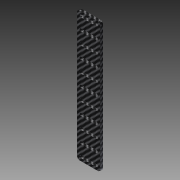
# Autodesk Inventor part: Kicker Plate
Saved by Autodesk Inventor 2015 (Build 190159000, 159)
## iProperties
Created: 2016-09-23
Part Number: Kicker Plate
Material: Generic
Document SubType Name: Modeling
Designer: James Yelland
Density: 1 g/cm^3
Appearance: Default
Author: James Yelland
Autodesk Inventor part; units mm, degrees
ref_plane "YZ Plane" through (0, 0, 0) normal (1, 0, 0) x (0, 1, 0)
ref_plane "XZ Plane" through (0, 0, 0) normal (0, 1, 0) x (-1, 0, 0)
ref_plane "XY Plane" through (0, 0, 0) normal (0, 0, 1) x (1, 0, 0)
sketch "Sketch1" plane through (0, 0, 0) normal (0, 1, 0) x (-1, 0, 0)
  line L0 (-9, 48) -> (-9, -48)
  line L1 (-7, -50) -> (7, -50)
  line L2 (9, -48) -> (9, 48)
  line L3 (7, 50) -> (-7, 50)
  line L4 (-9, 50) -> (9, -50) construction
  line L5 (-9, -50) -> (9, 50) construction
  arc A0 (9, 48) -> (7, 50) centre (7, 48) ccw
  arc A1 (-7, 50) -> (-9, 48) centre (-7, 48) ccw
  arc A2 (-9, -48) -> (-7, -50) centre (-7, -48) ccw
  arc A3 (7, -50) -> (9, -48) centre (7, -48) ccw
  line L6 (-7, 47) -> (-7, 47)
  line L7 (-6, 46) -> (6, 46)
  line L8 (7, 47) -> (7, 47)
  line L9 (6, 48) -> (-6, 48)
  arc A4 (7, 47) -> (6, 48) centre (6, 47) ccw
  arc A5 (6, 46) -> (7, 47) centre (6, 47) ccw
  arc A6 (-6, 48) -> (-7, 47) centre (-6, 47) ccw
  arc A7 (-7, 47) -> (-6, 46) centre (-6, 47) ccw
  line L10 (-7, 37.6) -> (-7, 37.6)
  line L11 (-6, 36.6) -> (6, 36.6)
  line L12 (7, 37.6) -> (7, 37.6)
  line L13 (6, 38.6) -> (-6, 38.6)
  arc A8 (7, 37.6) -> (6, 38.6) centre (6, 37.6) ccw
  arc A9 (6, 36.6) -> (7, 37.6) centre (6, 37.6) ccw
  arc A10 (-6, 38.6) -> (-7, 37.6) centre (-6, 37.6) ccw
  arc A11 (-7, 37.6) -> (-6, 36.6) centre (-6, 37.6) ccw
  line L14 (-7, 28.2) -> (-7, 28.2)
  line L15 (-6, 27.2) -> (6, 27.2)
  line L16 (7, 28.2) -> (7, 28.2)
  line L17 (6, 29.2) -> (-6, 29.2)
  arc A12 (7, 28.2) -> (6, 29.2) centre (6, 28.2) ccw
  arc A13 (6, 27.2) -> (7, 28.2) centre (6, 28.2) ccw
  arc A14 (-6, 29.2) -> (-7, 28.2) centre (-6, 28.2) ccw
  arc A15 (-7, 28.2) -> (-6, 27.2) centre (-6, 28.2) ccw
  line L18 (-7, 18.8) -> (-7, 18.8)
  line L19 (-6, 17.8) -> (6, 17.8)
  line L20 (7, 18.8) -> (7, 18.8)
  line L21 (6, 19.8) -> (-6, 19.8)
  arc A16 (7, 18.8) -> (6, 19.8) centre (6, 18.8) ccw
  arc A17 (6, 17.8) -> (7, 18.8) centre (6, 18.8) ccw
  arc A18 (-6, 19.8) -> (-7, 18.8) centre (-6, 18.8) ccw
  arc A19 (-7, 18.8) -> (-6, 17.8) centre (-6, 18.8) ccw
  line L22 (-7, 9.4) -> (-7, 9.4)
  line L23 (-6, 8.4) -> (6, 8.4)
  line L24 (7, 9.4) -> (7, 9.4)
  line L25 (6, 10.4) -> (-6, 10.4)
  arc A20 (7, 9.4) -> (6, 10.4) centre (6, 9.4) ccw
  arc A21 (6, 8.4) -> (7, 9.4) centre (6, 9.4) ccw
  arc A22 (-6, 10.4) -> (-7, 9.4) centre (-6, 9.4) ccw
  arc A23 (-7, 9.4) -> (-6, 8.4) centre (-6, 9.4) ccw
  line L26 (-7, 0) -> (-7, 0)
  line L27 (-6, -1) -> (6, -1)
  line L28 (7, 0) -> (7, 0)
  line L29 (6, 1) -> (-6, 1)
  arc A24 (7, 0) -> (6, 1) centre (6, 0) ccw
  arc A25 (6, -1) -> (7, 0) centre (6, 0) ccw
  arc A26 (-6, 1) -> (-7, 0) centre (-6, 0) ccw
  arc A27 (-7, 0) -> (-6, -1) centre (-6, 0) ccw
  line L30 (-7, -9.4) -> (-7, -9.4)
  line L31 (-6, -10.4) -> (6, -10.4)
  line L32 (7, -9.4) -> (7, -9.4)
  line L33 (6, -8.4) -> (-6, -8.4)
  arc A28 (7, -9.4) -> (6, -8.4) centre (6, -9.4) ccw
  arc A29 (6, -10.4) -> (7, -9.4) centre (6, -9.4) ccw
  arc A30 (-6, -8.4) -> (-7, -9.4) centre (-6, -9.4) ccw
  arc A31 (-7, -9.4) -> (-6, -10.4) centre (-6, -9.4) ccw
  line L34 (-7, -18.8) -> (-7, -18.8)
  line L35 (-6, -19.8) -> (6, -19.8)
  line L36 (7, -18.8) -> (7, -18.8)
  line L37 (6, -17.8) -> (-6, -17.8)
  arc A32 (7, -18.8) -> (6, -17.8) centre (6, -18.8) ccw
  arc A33 (6, -19.8) -> (7, -18.8) centre (6, -18.8) ccw
  arc A34 (-6, -17.8) -> (-7, -18.8) centre (-6, -18.8) ccw
  arc A35 (-7, -18.8) -> (-6, -19.8) centre (-6, -18.8) ccw
  line L38 (-7, -28.2) -> (-7, -28.2)
  line L39 (-6, -29.2) -> (6, -29.2)
  line L40 (7, -28.2) -> (7, -28.2)
  line L41 (6, -27.2) -> (-6, -27.2)
  arc A36 (7, -28.2) -> (6, -27.2) centre (6, -28.2) ccw
  arc A37 (6, -29.2) -> (7, -28.2) centre (6, -28.2) ccw
  arc A38 (-6, -27.2) -> (-7, -28.2) centre (-6, -28.2) ccw
  arc A39 (-7, -28.2) -> (-6, -29.2) centre (-6, -28.2) ccw
  line L42 (-7, -37.6) -> (-7, -37.6)
  line L43 (-6, -38.6) -> (6, -38.6)
  line L44 (7, -37.6) -> (7, -37.6)
  line L45 (6, -36.6) -> (-6, -36.6)
  arc A40 (7, -37.6) -> (6, -36.6) centre (6, -37.6) ccw
  arc A41 (6, -38.6) -> (7, -37.6) centre (6, -37.6) ccw
  arc A42 (-6, -36.6) -> (-7, -37.6) centre (-6, -37.6) ccw
  arc A43 (-7, -37.6) -> (-6, -38.6) centre (-6, -37.6) ccw
  line L46 (-7, -47) -> (-7, -47)
  line L47 (-6, -48) -> (6, -48)
  line L48 (7, -47) -> (7, -47)
  line L49 (6, -46) -> (-6, -46)
  arc A44 (7, -47) -> (6, -46) centre (6, -47) ccw
  arc A45 (6, -48) -> (7, -47) centre (6, -47) ccw
  arc A46 (-6, -46) -> (-7, -47) centre (-6, -47) ccw
  arc A47 (-7, -47) -> (-6, -48) centre (-6, -47) ccw
  point P0 (0, 0)
  point P1 (-7, 46)
  point P2 (7, 38.6)
  point P3 (-7, 38.6)
  point P4 (-7, 36.6)
  point P5 (7, 29.2)
  point P6 (-7, 29.2)
  point P7 (-7, 27.2)
  point P8 (7, 19.8)
  point P9 (-7, 19.8)
  point P10 (-7, 17.8)
  point P11 (7, 10.4)
  point P12 (-7, 10.4)
  point P13 (-7, 8.4)
  point P14 (7, 1)
  point P15 (-7, 1)
  point P16 (-7, -1)
  point P17 (7, -8.4)
  point P18 (-7, -8.4)
  point P19 (-7, -10.4)
  point P20 (7, -17.8)
  point P21 (-7, -17.8)
  point P22 (-7, -19.8)
  point P23 (7, -27.2)
  point P24 (-7, -27.2)
  point P25 (-7, -29.2)
  point P26 (7, -36.6)
  point P27 (-7, -36.6)
  point P28 (-7, -38.6)
  point P29 (7, -46)
  point P30 (-7, -46)
  point P31 (-7, -48)
  dimension "d0" = 100
  dimension "d1" = 18
  dimension "d2" = 2
  dimension "d3" = 2
  dimension "d4" = 1
  dimension "d5" = 1
  dimension "d8" = 9.4
  constraints: 100 end point, 96 point on circle, 74 point on line, 48 centre point, 16 tangent, 5 equal radius, 4 perpendicular, 3 vertical, 2 midpoint, 2 parallel, 230 other
  measures "d0" distance of L4.start L5.start
  measures "d1" distance of L4.end L5.start
  measures "d2" radius of A0
  measures "d3" distance of A1.centre point (-7, 46)
  measures "d4" radius of A4
  measures "d5" radius of A6
  measures "d8" distance of L7.end L11.end
extrude "Extrusion1" add sketch "Sketch1" along normal blind 2
body "Solid1"
